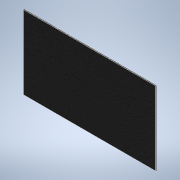
# Autodesk Inventor part: vidrio_ir
Saved by Autodesk Inventor 2021 (Build 250183000, 183)
## iProperties
Created: 2021-11-08
Part Number: vidrio_ir
Material: Genérico
Document SubType Name: Modeling
Designer: arthu
Density: 1 g/cm^3
Appearance: Negro
Author: arthu
Autodesk Inventor part; units mm, degrees
ref_plane "YZ Plane" through (0, 0, 0) normal (1, 0, 0) x (0, 1, 0)
ref_plane "XZ Plane" through (0, 0, 0) normal (0, 1, 0) x (-1, 0, 0)
ref_plane "XY Plane" through (0, 0, 0) normal (0, 0, 1) x (1, 0, 0)
sketch "Boceto1" plane through (0, 0, 0) normal (0, 0, 1) x (1, 0, 0)
  line L0 (260, -145) -> (-260, -145)
  line L1 (-260, -145) -> (-260, 145)
  line L2 (-260, 145) -> (260, 145)
  line L3 (260, 145) -> (260, -145)
  line L4 (260, -145) -> (-260, 145) construction
  line L5 (-260, -145) -> (260, 145) construction
  point P0 (0, 0)
  dimension "d0" = 520
  dimension "d1" = 290
  constraints: 12 end point, 2 midpoint, 2 parallel, 1 horizontal, 1 perpendicular
  measures "d0" distance of L1.end L2.end
  measures "d1" distance of L0.end L1.end
extrude "Extrusión1" add sketch "Boceto1" along normal blind 4
chamfer "Chaflán1" distance 0.8 angle 45 8 edges at (0, 145, 4) (0, 145, 0) (-260, 0, 4) (-260, 0, 0) (260, 0, 4) (260, 0, 0) (0, -145, 0) (0, -145, 4)
